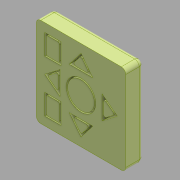
# Autodesk Inventor part: Part2
Saved by Autodesk Inventor 2016 (Build 200138000, 138)
## iProperties
Created: 2016-08-15
Part Number: Part2
Material: Generic
Document SubType Name: Modeling
Designer: ADMIN
Density: 1 g/cm^3
Appearance: Zinc Chromate 2
Author: ADMIN
Autodesk Inventor part; units mm, degrees
ref_plane "YZ Plane" through (0, 0, 0) normal (1, 0, 0) x (0, 1, 0)
ref_plane "XZ Plane" through (0, 0, 0) normal (0, 1, 0) x (-1, 0, 0)
ref_plane "XY Plane" through (0, 0, 0) normal (0, 0, 1) x (1, 0, 0)
sketch "Sketch1" plane through (0, 0, 0) normal (0, 1, 0) x (-1, 0, 0)
  circle A0 centre (0, 0) radius 15
  line L0 (0, -25) -> (10, -25)
  line L1 (0, -25) -> (-10, -25)
  line L2 (-10, -25) -> (0, -38)
  line L3 (0, -38) -> (10, -25)
  line L4 (25, 0) -> (25, 10)
  line L5 (25, 0) -> (25, -10)
  line L6 (25, -10) -> (38, 0)
  line L7 (38, 0) -> (25, 10)
  line L8 (0, 25) -> (-10, 25)
  line L9 (0, 25) -> (10, 25)
  line L10 (10, 25) -> (0, 38)
  line L11 (0, 38) -> (-10, 25)
  line L12 (-25, 0) -> (-25, -10)
  line L13 (-25, 0) -> (-25, 10)
  line L14 (-25, 10) -> (-38, 0)
  line L15 (-38, 0) -> (-25, -10)
  line L16 (38.9602, 38.9602) -> (23.9602, 38.9602)
  line L17 (23.9602, 38.9602) -> (23.9602, 18.9602)
  line L18 (23.9602, 18.9602) -> (38.9602, 18.9602)
  line L19 (38.9602, 18.9602) -> (38.9602, 38.9602)
  line L20 (38.9602, -38.9602) -> (23.9602, -38.9602)
  line L21 (23.9602, -38.9602) -> (23.9602, -18.9602)
  line L22 (23.9602, -18.9602) -> (38.9602, -18.9602)
  line L23 (38.9602, -18.9602) -> (38.9602, -38.9602)
  line L24 (40.4602, -40.4602) -> (22.4602, -40.4602)
  line L25 (22.4602, -40.4602) -> (22.4602, -17.4602)
  line L26 (22.4602, -17.4602) -> (40.4602, -17.4602)
  line L27 (40.4602, -17.4602) -> (40.4602, -40.4602)
  line L28 (40.4602, 40.4602) -> (22.4602, 40.4602)
  line L29 (22.4602, 40.4602) -> (22.4602, 17.4602)
  line L30 (22.4602, 17.4602) -> (40.4602, 17.4602)
  line L31 (40.4602, 17.4602) -> (40.4602, 40.4602)
  line L32 (0, 40.4602) -> (13.0463, 23.5)
  line L33 (13.0463, 23.5) -> (0, 23.5)
  line L34 (0, 23.5) -> (-13.0463, 23.5)
  line L35 (-13.0463, 23.5) -> (0, 40.4602)
  line L36 (13.0463, -23.5) -> (0, -23.5)
  line L37 (0, -23.5) -> (-13.0463, -23.5)
  line L38 (-13.0463, -23.5) -> (0, -40.4602)
  line L39 (0, -40.4602) -> (13.0463, -23.5)
  line L40 (23.5, 13.0463) -> (23.5, 0)
  line L41 (23.5, 0) -> (23.5, -13.0463)
  line L42 (23.5, -13.0463) -> (40.4602, 0)
  line L43 (40.4602, 0) -> (23.5, 13.0463)
  line L44 (-23.5, -13.0463) -> (-23.5, 0)
  line L45 (-23.5, 0) -> (-23.5, 13.0463)
  line L46 (-23.5, 13.0463) -> (-40.4602, 0)
  line L47 (-40.4602, 0) -> (-23.5, -13.0463)
  circle A1 centre (0, 0) radius 16.4012
  line L48 (0, 50) -> (50, 50)
  line L49 (50, 50) -> (50, -50)
  line L50 (50, -50) -> (-50, -50)
  line L51 (-50, -50) -> (-50, 50)
  line L52 (-50, 50) -> (0, 50)
  dimension "d1" = 10
  dimension "d2" = 10
  dimension "d5" = 360
  dimension "d7" = 15
  dimension "d8" = 20
  dimension "d9" = 15
  dimension "d10" = 20
  dimension "d11" = 1.5
  dimension "d12" = 1.5
  dimension "d13" = 1.5
  dimension "d14" = 1.5
  dimension "d15" = 1.5
  dimension "d16" = 1.5
  dimension "d17" = 1.4012
  dimension "d18" = 50
  dimension "d19" = 100
  dimension "d20" = 100
  dimension "d21" = 100
  constraints: 106 end point, 8 parallel, 6 perpendicular, 5 horizontal, 2 centre point, 1 coincident, 1 point on line, 51 other
  measures "d1" distance of L0.start L0.end
  measures "d2" distance of L0.start L1.end
  measures "d7" distance of L18.end L17.end
  measures "d8" distance of L17.end L16.end
  measures "d9" distance of L21.end L22.end
  measures "d10" distance of L20.end L21.end
  measures "d11" distance between parallel lines of L23 L27
  measures "d12" distance between parallel lines of L19 L31
  measures "d13" distance between parallel lines of L10 L32
  measures "d14" distance between parallel lines of L3 L39
  measures "d15" distance between parallel lines of L7 L43
  measures "d16" distance between parallel lines of L15 L47
  measures "d17" radial gap between concentric circles of A0 A1
  measures "d18" distance of L48.start L48.end
  measures "d19" distance of L48.end L49.end
  measures "d20" distance of L49.end L50.end
  measures "d21" distance of L50.end L51.end
extrude "Extrusion1" add sketch "Sketch1" along normal blind 20
fillet "Fillet1" radius 2 1 edges at (-23.9602, 10, 38.9602)
fillet "Fillet2" radius 2 1 edges at (-38.9602, 10, 38.9602)
fillet "Fillet3" radius 2 1 edges at (-23.9602, 10, 18.9602)
fillet "Fillet4" radius 2 1 edges at (-38.9602, 10, 18.9602)
fillet "Fillet5" radius 2 1 edges at (-38, 10, 0)
fillet "Fillet6" radius 2 1 edges at (-25, 10, 10)
fillet "Fillet7" radius 2 1 edges at (-25, 10, -10)
fillet "Fillet8" radius 2 1 edges at (-38.9602, 10, -18.9602)
fillet "Fillet9" radius 2 1 edges at (-38.9602, 10, -38.9602)
fillet "Fillet10" radius 2 1 edges at (-23.9602, 10, -38.9602)
fillet "Fillet11" radius 2 1 edges at (-23.9602, 10, -18.9602)
fillet "Fillet12" radius 2 1 edges at (-10, 10, -25)
fillet "Fillet13" radius 2 1 edges at (10, 10, -25)
fillet "Fillet14" radius 2 1 edges at (0, 10, -38)
fillet "Fillet15" radius 2 1 edges at (25, 10, 10)
fillet "Fillet16" radius 2 1 edges at (25, 10, -10)
fillet "Fillet17" radius 2 1 edges at (38, 10, 0)
fillet "Fillet18" radius 2 1 edges at (-10, 10, 25)
fillet "Fillet19" radius 2 1 edges at (10, 10, 25)
fillet "Fillet20" radius 2 1 edges at (0, 10, 38)
fillet "Fillet21" radius 2 1 edges at (15, 20, 0)
fillet "Fillet22" radius 2 8 edges at (-38.9602, 20, 28.9602) (-38.3744, 20, 38.3744) (-31.4602, 20, 38.9602) (-24.546, 20, 38.3744) (-23.9602, 20, 28.9602) (-24.546, 20, 19.546) (-31.4602, 20, 18.9602) (-38.3744, 20, 19.546)
fillet "Fillet23" radius 2 6 edges at (-26.1165, 20, 7.7325) (-32.0793, 20, 4.5544) (-36.7198, 20, 0) (-32.0793, 20, -4.5544) (-26.1165, 20, -7.7325) (-25, 20, 0)
fillet "Fillet24" radius 2 8 edges at (-31.4602, 20, -18.9602) (-24.546, 20, -19.546) (-23.9602, 20, -28.9602) (-24.546, 20, -38.3744) (-31.4602, 20, -38.9602) (-38.3744, 20, -38.3744) (-38.9602, 20, -28.9602) (-38.3744, 20, -19.546)
fillet "Fillet25" radius 2 6 edges at (-4.5544, 20, -32.0793) (-7.7325, 20, -26.1165) (0, 20, -25) (7.7325, 20, -26.1165) (4.5544, 20, -32.0793) (0, 20, -36.7198)
fillet "Fillet26" radius 2 6 edges at (0, 20, 25) (-7.7325, 20, 26.1165) (-4.5544, 20, 32.0793) (0, 20, 36.7198) (4.5544, 20, 32.0793) (7.7325, 20, 26.1165)
fillet "Fillet27" radius 2 6 edges at (25, 20, 0) (26.1165, 20, 7.7325) (32.0793, 20, 4.5544) (36.7198, 20, 0) (32.0793, 20, -4.5544) (26.1165, 20, -7.7325)
fillet "Fillet28" radius 2 1 edges at (16.4012, 20, 0)
fillet "Fillet29" radius 1 4 edges at (-40.4602, 20, 28.9602) (-31.4602, 20, 17.4602) (-22.4602, 20, 28.9602) (-31.4602, 20, 40.4602)
fillet "Fillet30" radius 1 3 edges at (-31.9801, 20, -6.5231) (-23.5, 20, 0) (-31.9801, 20, 6.5231)
fillet "Fillet31" radius 1 4 edges at (-31.4602, 20, -17.4602) (-40.4602, 20, -28.9602) (-31.4602, 20, -40.4602) (-22.4602, 20, -28.9602)
fillet "Fillet32" radius 1 3 edges at (-6.5231, 20, -31.9801) (0, 20, -23.5) (6.5231, 20, -31.9801)
fillet "Fillet33" radius 1 3 edges at (0, 20, 23.5) (6.5231, 20, 31.9801) (-6.5231, 20, 31.9801)
fillet "Fillet34" radius 1 3 edges at (23.5, 20, 0) (31.9801, 20, 6.5231) (31.9801, 20, -6.5231)
fillet "Fillet35" radius 5 3 edges at (-50, 10, 50) (50, 10, -50) (50, 10, 50)
fillet "Fillet36" radius 5 1 edges at (-50, 10, -50)
fillet "Fillet37" radius 5 8 edges at (-48.5355, 20, 48.5355) (0, 20, 50) (48.5355, 20, 48.5355) (50, 20, 0) (48.5355, 20, -48.5355) (0, 20, -50) (-48.5355, 20, -48.5355) (-50, 20, 0)
body "Solid1"
